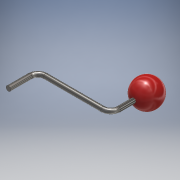
# Autodesk Inventor part: Poigner
Saved by Autodesk Inventor 2017 (Build 210142000, 142)
## iProperties
Part Number: Poigner
Material: Générique
Document SubType Name: Modeling
Designer: Adrien MARY
Density: 1 g/cm^3
Appearance: Par défaut
Author: Adrien MARY
Autodesk Inventor part; units mm, degrees
ref_plane "YZ Plane" through (0, 0, 0) normal (1, 0, 0) x (0, 1, 0)
ref_plane "XZ Plane" through (0, 0, 0) normal (0, 1, 0) x (-1, 0, 0)
ref_plane "XY Plane" through (0, 0, 0) normal (0, 0, 1) x (1, 0, 0)
sketch "Esquisse1" plane through (0, 0, 0) normal (0, 0, 1) x (1, 0, 0)
  line L0 (0, 0) -> (0, 27.5)
  line L1 (10, 37.5) -> (83, 37.5)
  line L2 (93, 47.5) -> (93, 83.5)
  arc A0 (10, 37.5) -> (0, 27.5) centre (10, 27.5) ccw
  arc A1 (83, 37.5) -> (93, 47.5) centre (83, 47.5) ccw
  dimension "d0" = 93
  dimension "d1" = 37.5
  dimension "d2" = 46
  dimension "d3" = 10
  constraints: 6 end point, 4 point on circle, 4 tangent, 2 centre point, 2 vertical, 1 equal radius, 1 horizontal
  measures "d0" distance between parallel lines of L2 L0
  measures "d1" distance from line of L0.start L1
  measures "d2" distance from line of L2.end L1
  measures "d3" radius of A0
sketch "Esquisse2" plane through (0, 0, 0) normal (0, 1, 0) x (-1, 0, 0)
  circle A0 centre (0, 0) radius 3
  dimension "d4" = 6
  constraints: 1 centre point, 1 coincident
  measures "d4" diameter of A0
sweep "Balayage1" add profiles "Esquisse2" path "Esquisse1"
sketch "Esquisse3" plane through (93, 83.5, 0) normal (0, 1, 0) x (1, 0, 0)
  arc A0 (17.25, 0) -> (-17.25, 0) centre (0, 0) ccw
  circle A1 centre (0, 0) radius 3 construction
  line L0 (17.25, 0) -> (-17.25, 0)
  line L1 (-83, 3) -> (-10, 3) projected
  point P0 (-93, 0)
  dimension "d7" = 34.5
  constraints: 2 coincident, 2 end point, 2 point on circle, 1 centre point, 1 midpoint, 1 parallel
  measures "d7" diameter of A0
revolve "Révolution1" add sketch "Esquisse3" angle 360 about axis through (110.25, 83.5, 0) along (-1, 0, 0) separate body
equation "\"nombredor\" = 1.61803"
equation "\"pi\" = 3.141593"
